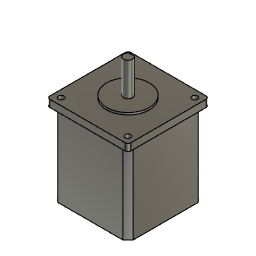
Motor assembly (Autodesk Fusion 360 archive; units mm, degrees)
design "nema_23"
Autodesk Fusion 360 part; units mm, degrees
sketch "Sketch1" plane through (0, 0, 0) normal (0, 0, 1) x (1, 0, 0)
  circle A0 centre (0, 0) radius 3.175
  line L0 (-1.9572, 2.5) -> (1.9572, 2.5)
  line L1 (-23.5, 23.5) -> (23.5, 23.5) construction
  line L2 (23.5, 23.5) -> (23.5, -23.5) construction
  line L3 (23.5, -23.5) -> (-23.5, -23.5) construction
  line L4 (-23.5, -23.5) -> (-23.5, 23.5) construction
  line L5 (-28.5, 28.5) -> (28.5, 28.5)
  line L6 (28.5, 28.5) -> (28.5, -28.5)
  line L7 (28.5, -28.5) -> (-28.5, -28.5)
  line L8 (-28.5, -28.5) -> (-28.5, 28.5)
  line L9 (-23.5, 23.5) -> (23.5, -23.5) construction
  line L10 (28.5, 28.5) -> (-28.5, -28.5) construction
  circle A1 centre (-23.5, 23.5) radius 2
  circle A2 centre (-23.5, -23.5) radius 2
  circle A3 centre (23.5, -23.5) radius 2
  circle A4 centre (23.5, 23.5) radius 2
  circle A5 centre (0, 0) radius 15
  dimension "d1" = 6.35
  dimension "d2" = 2.5
  dimension "d3" = 47
  dimension "d5" = 57
  dimension "d6" = 4
  dimension "d8" = 360
  dimension "d9" = 30
  constraint coincident A0.centre A5.centre
  constraint coincident A0 L0.start
  constraint coincident A0 L0.end
  constraint horizontal L0
  constraint horizontal L1
  constraint vertical L2
  constraint horizontal L3
  constraint vertical L4
  constraint horizontal L5
  constraint vertical L6
  constraint horizontal L7
  constraint vertical L8
  constraint equal L1 L4
  constraint equal L5 L8
  constraint midpoint L9 L10
  constraint midpoint L9 A0.centre
  constraint coincident L1.start L4.end
  constraint concentric A0 A5
  measures "d1" diameter of A0
  measures "d2" distance of A0.centre L0
  measures "d3" distance of L1.start L1.end
  measures "d5" distance of L5.start L5.end
  measures "d6" diameter of A1
  measures "d9" diameter of A5
extrude "Extrude1" add sketch "Sketch1" against normal blind 5 contours A0 L0 | A0 L0 | L5 L6 L7 L8 | A5
sketch "Sketch2" plane through (0, 0, -5) normal (0, 0, -1) x (1, 0, 0)
  circle A0 centre (-23.5, -23.5) radius 2
  circle A1 centre (-23.5, 23.5) radius 2
  circle A2 centre (23.5, 23.5) radius 2
  circle A3 centre (23.5, -23.5) radius 2
  line L0 (28.5, 28.5) -> (-28.5, 28.5)
  line L1 (-28.5, 28.5) -> (-28.5, -28.5)
  line L2 (-28.5, -28.5) -> (28.5, -28.5)
  line L3 (28.5, -28.5) -> (28.5, 28.5)
  line L4 (-28.5, -28.5) -> (28.5, 28.5) construction
  circle A4 centre (0, 0) radius 35
  line L5 (26.5, -26.5) -> (26.5, 26.5)
  line L6 (26.5, 26.5) -> (-26.5, 26.5)
  line L7 (-26.5, 26.5) -> (-26.5, -26.5)
  line L8 (-26.5, -26.5) -> (26.5, -26.5)
  dimension "d12" = 70
  dimension "d13" = -2
  constraint coincident L1.end L2.start
  constraint coincident L0.start L3.end
  constraint coincident A4.centre origin
  measures "d12" diameter of A4
extrude "Extrude2" add sketch "Sketch2" along normal blind 57 contours A0 A4 | A0 A1 A2 A3 A4 L5 L6 L7 L8 | A1 A4 | A3 A4 | A2 A4 picked at (-23.8415, -23.8801) picked at (-23.8415, 23.8801) picked at (23.863, -23.8578) picked at (23.863, 23.8578)
extrude "Extrude3" add sketch "Sketch1" along normal blind 25 contours A0 L0 picked at (0.6292, 0.6577)
extrude "Extrude4" add sketch "Sketch1" along normal blind 1.5 contours A5
fillet "Fillet1" radius 2 4 edges at (-28.5, 28.5, -2.5) (28.5, 28.5, -2.5) (28.5, -28.5, -2.5) (-28.5, -28.5, -2.5)
